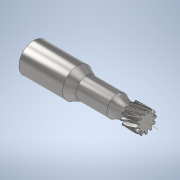
# Autodesk Inventor part: Валл быстроходный
Saved by Autodesk Inventor 2021 (Build 250183000, 183)
## iProperties
Created: 2023-03-09
Part Number: Валл быстроходный
Material: Сталь, углеродистая
Document SubType Name: Modeling
Designer: gdevc
Density: 7.85 g/cm^3
Appearance: С умеренной полировкой
Mass: 848.958 g
Surface Area: 271.138 cm^2
Volume: 108.148 cm^3
Author: gdevc
Autodesk Inventor part; units mm, degrees
ref_plane "YZ Plane" through (0, 0, 0) normal (1, 0, 0) x (0, 1, 0)
ref_plane "XZ Plane" through (0, 0, 0) normal (0, 1, 0) x (-1, 0, 0)
ref_plane "XY Plane" through (0, 0, 0) normal (0, 0, 1) x (1, 0, 0)
sketch "Эскиз1" plane through (0, 0, 0) normal (0, 0, 1) x (1, 0, 0)
  line L0 (0, 14) -> (0, 21)
  line L1 (0, 21) -> (62.305, 21)
  line L2 (62.305, 21) -> (75.172, 15)
  line L3 (75.172, 15) -> (119.367, 15)
  line L4 (160.55, 15.6) -> (160.55, 0)
  line L5 (160.55, 0) -> (0, 0) construction
  line L6 (0, 14) -> (62.305, 14)
  line L7 (62.305, 14) -> (62.305, 0)
  line L8 (62.305, 14) -> (70.3879, 0)
  line L9 (70.3879, 0) -> (62.305, 0)
  line L10 (70.3879, 0) -> (160.55, 0)
  line L11 (160.55, 15.6) -> (138.55, 15.6)
  line L12 (138.55, 15.6) -> (138.55, 10.1)
  arc A0 (119.367, 15) -> (138.55, 10.1) centre (138.55, 50.1) ccw
  dimension "d1" = 42
  dimension "d2" = 30
  dimension "d3" = 28
  dimension "d4" = 62.305
  dimension "d5" = 25
  dimension "d14" = 30
  dimension "d15" = 31.2
  dimension "d27" = 22
  dimension "d30" = 20.2
  dimension "d31" = 40
  dimension "d32" = 85.378
  constraints: 26 end point, 4 perpendicular, 3 horizontal, 3 point on line, 2 point on circle, 2 vertical, 2 vertical alignment, 1 centre point, 1 collinear
  measures "d1" diameter of L1 L5
  measures "d2" angle of L7 L8
  measures "d3" diameter of L6 L5
  measures "d4" distance of L0.start L6.end
  measures "d5" angle of L3 L2
  measures "d14" diameter of L3 L5
  measures "d15" diameter of L11 L5
  measures "d27" distance of L4.start L11.end
  measures "d30" diameter of L12.end L5
  measures "d31" radius of A0
  measures "d32" distance from line of L4 L2.end
revolve "Вращение1" add sketch "Эскиз1" angle 360 about axis through (160.55, 0, 0) along (-1, 0, 0) contours L0 L1 L2 L3 A0 L12 L11 L4 L10 L8 L6
sketch "Эскиз2" plane through (0, 0, 0) normal (-1, 0, 0) x (0, 0, 1)
  circle A0 centre (0, 0) radius 14 projected
  line L0 (-4, 17.6) -> (4, 17.6)
  line L1 (4, 17.6) -> (4, 10)
  line L2 (4, 10) -> (-4, 10)
  line L3 (-4, 10) -> (-4, 17.6)
  point P0 (0, 17.6)
  point P1 (-4, 13.4164)
  point P2 (4, 13.4164)
  dimension "d8" = 8
  dimension "d9" = 7.6
  dimension "d11" = 4
  constraints: 8 end point, 2 parallel, 1 horizontal, 1 midpoint, 1 perpendicular, 1 vertical alignment
  measures "d8" distance of L0.start L0.end
  measures "d9" distance between parallel lines of L2 L0
  measures "d11" distance edge to line of A0 L2
extrude "Выдавливание1" cut sketch "Эскиз2" against normal blind 62.305 contours A0 L3 L0 L1
spur gear teeth "Цилиндрическое зубчатое зацепление1" teeth 12 pitch diameter 25.2 tip diameter 29.2 root diameter 20.2 face width 22 helix angle 17.753 hand left trims to tip circle yes start plane through (160.55, 0, 0) normal (1, 0, 0) x (0, 1, 0)
